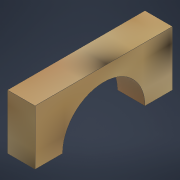
# Autodesk Inventor part: 110033226_ipt_09_窗戶圓拱
Saved by Autodesk Inventor 2022 (Build 260153000, 153)
## iProperties
Created: 2022-06-22
Part Number: 110033226_ipt_09_窗戶圓拱
Material: 一般
Document SubType Name: Modeling
Designer: User
Density: 1 g/cm^3
Appearance: 預設
Author: User
Autodesk Inventor part; units mm, degrees
ref_plane "YZ Plane" through (0, 0, 0) normal (1, 0, 0) x (0, 1, 0)
ref_plane "XZ Plane" through (0, 0, 0) normal (0, 1, 0) x (-1, 0, 0)
ref_plane "XY Plane" through (0, 0, 0) normal (0, 0, 1) x (1, 0, 0)
sketch "草圖1" plane through (0, 0, 0) normal (0, 1, 0) x (-1, 0, 0)
  line L0 (2.5, 12.5) -> (-2.5, 12.5)
  line L1 (-2.5, 12.5) -> (-2.5, -12.5)
  line L2 (-2.5, -12.5) -> (2.5, -12.5)
  line L3 (2.5, -12.5) -> (2.5, 12.5)
  circle A0 centre (0, 10) radius 1.7
  circle A1 centre (0, 5) radius 1.7
  circle A2 centre (0, 0) radius 1.7
  circle A3 centre (0, -5) radius 1.7
  circle A4 centre (0, -10) radius 1.7
  point P0 (0, 0)
  point P1 (2.5, 0)
  point P2 (0, 12.5)
  dimension "d0" = 5
  dimension "d1" = 25
  dimension "d2" = 3.4
  dimension "d3" = 2.5
  dimension "d4" = 2.5
  dimension "d7" = 5
  constraints: 8 end point, 5 centre point, 2 midpoint, 2 parallel, 1 horizontal, 1 horizontal alignment, 1 perpendicular, 1 vertical, 1 vertical alignment, 8 other
  measures "d0" distance of L2.end L1.end
  measures "d1" distance of L1.end L0.end
  measures "d2" diameter of A0
  measures "d3" distance from line of L0 A0.centre
  measures "d4" distance from line of L1 A0.centre
  measures "d7" distance of A0.centre A1.centre
sketch "草圖2" plane through (0, 0, 0) normal (1, 0, 0) x (0, 1, 0)
  line L0 (0, -12.5) -> (0, 12.5) projected
  circle A0 centre (0, 0) radius 7.5
  line L1 (0, 12.5) -> (10, 12.5)
  line L2 (10, 12.5) -> (10, -12.5)
  line L3 (10, -12.5) -> (0, -12.5)
  point P0 (0, 10)
  point P1 (0, 5)
  point P2 (0, -5)
  point P3 (0, -10)
  point P4 (0, 7.5)
  point P5 (0, -7.5)
  dimension "d12" = 15
  dimension "d13" = 10
  constraints: 6 end point, 2 perpendicular, 1 centre point, 1 coincident, 1 vertical
  measures "d12" diameter of A0
  measures "d13" distance of L2.end L0.start
extrude "擠出1" add sketch "草圖2" along normal mid plane 5 contours L0 A0 L1 L2 L3
extrude "擠出2" cut sketch "草圖1" along normal blind 1.5 contours A0 | A4
